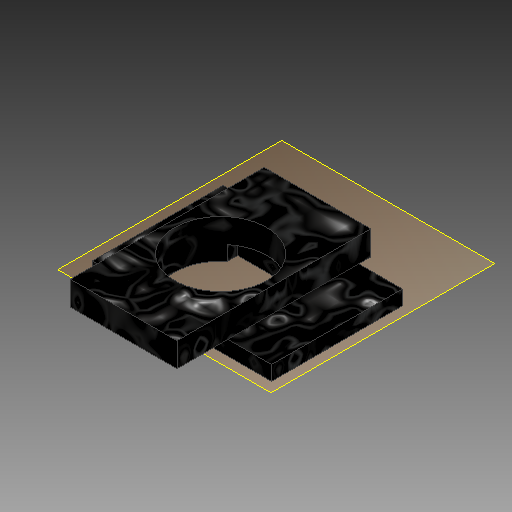
# Autodesk Inventor part: 04_LED_Holder
Saved by Autodesk Inventor 2019 (Build 230136000, 136)
## iProperties
Created: 2016-11-08
Part Number: 04_LED_Holder
Material: Generisch
Document SubType Name: Modeling
Designer: Bene
Density: 1 g/cm^3
Appearance: Schwarz
Author: Bene
Autodesk Inventor part; units mm, degrees
ref_plane "YZ Plane" through (0, 0, 0) normal (1, 0, 0) x (0, 1, 0)
ref_plane "XZ Plane" through (0, 0, 0) normal (0, 1, 0) x (-1, 0, 0)
ref_plane "Arbeitsebene1" through (0, 0, 0) normal (0, 0, 1) x (1, 0, 0)
sketch "Skizze1" plane through (0, 0, 0) normal (0, 0, 1) x (1, 0, 0)
  line L0 (26, 19) -> (14, 19) projected
  line L1 (14, 19) -> (14, 0) projected
  line L2 (14, 0) -> (26, 0) projected
  line L3 (26, 0) -> (26, 19) projected
  line L4 (0, 0) -> (40, 0) projected
  line L5 (40, 0) -> (40, 42) projected
  line L6 (0, 42) -> (40, 42) projected
  line L7 (0, 0) -> (0, 42) projected
  line L8 (40, 0) -> (3, 0)
  line L9 (3, 0) -> (3, 27)
  line L10 (3, 27) -> (40, 27)
  line L11 (40, 27) -> (40, 0)
  dimension "d0" = 37
  dimension "d1" = 27
  constraints: 8 end point, 2 parallel, 1 horizontal, 1 perpendicular
  measures "d0" distance of L9.end L10.end
  measures "d1" distance of L8.end L9.end
extrude "Extrusion1" add sketch "Skizze1" along normal blind 3 contours L0 L1 L4 L9 L10 L5 L3
sketch "Skizze2" plane through (0, 0, 3) normal (0, 0, 1) x (1, 0, 0)
  line L0 (14, 0) -> (14, 19) projected
  line L1 (14, 19) -> (26, 19) projected
  line L2 (26, 19) -> (26, 0) projected
  line L3 (26, 0) -> (40, 0) projected
  line L4 (40, 0) -> (40, 27) projected
  line L5 (40, 27) -> (3, 27) projected
  line L6 (3, 27) -> (3, 0) projected
  line L7 (3, 0) -> (14, 0) projected
  line L8 (9, 29.5) -> (31, 29.5)
  line L9 (31, 29.5) -> (31, -10.5)
  line L10 (31, -10.5) -> (9, -10.5)
  line L11 (9, -10.5) -> (9, 29.5)
  line L12 (9, 29.5) -> (31, -10.5) construction
  line L13 (31, 29.5) -> (9, -10.5) construction
  point P0 (0, 0)
  point P1 (20, 9.5)
  dimension "d4" = 22
  dimension "d5" = 40
  constraints: 12 end point, 2 midpoint, 2 parallel, 1 horizontal, 1 perpendicular
  measures "d4" distance of L9.end L10.end
  measures "d5" distance of L8.end L9.end
extrude "Extrusion2" add sketch "Skizze2" along normal blind 5 contours L7 L11 L5 L9 L3 L2 L1 L0 | L0 L1 L2 L3 L9 L10 L11 L7 | L11 L8 L9 L5
sketch "Skizze3" plane through (0, 0, 8) normal (0, 0, 1) x (1, 0, 0)
  line L0 (14, 0) -> (14, 19) projected
  line L1 (14, 19) -> (26, 19) projected
  line L2 (26, 19) -> (26, 0) projected
  line L3 (14, 0) -> (26, 0) projected
  circle A0 centre (20, 9.5) radius 9.5
  point P0 (0, 0)
  constraints: 1 centre point, 1 tangent
ref_plane "Arbeitsebene2" through (0, 0, 0) normal (0, 0, 1) x (1, 0, 0)
extrude "Extrusion3" cut sketch "Skizze3" against normal up to surface (8 mm away) contours A0 L0 | L0 A0 L2 | L2 A0
